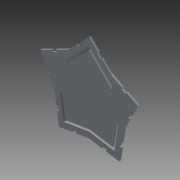
# Autodesk Inventor part: Star Base
Saved by Autodesk Inventor 2015 (Build 190159000, 159)
## iProperties
Created: 2018-03-07
Part Number: Star Base
Material: Generic
Document SubType Name: Modeling
Designer: Administrator
Density: 1 g/cm^3
Appearance: Default
Author: Administrator
Autodesk Inventor part; units mm, degrees
ref_plane "YZ Plane" through (0, 0, 0) normal (1, 0, 0) x (0, 1, 0)
ref_plane "XZ Plane" through (0, 0, 0) normal (0, 1, 0) x (-1, 0, 0)
ref_plane "XY Plane" through (0, 0, 0) normal (0, 0, 1) x (1, 0, 0)
sketch "Sketch1" plane through (0, 0, 0) normal (0, 0, 1) x (1, 0, 0)
  circle A0 centre (0, 0) radius 63.5 construction
  circle A1 centre (0, 0) radius 88.9 construction
  line L0 (0, 88.9) -> (-37.3244, 51.3726)
  line L1 (-37.3244, 51.3726) -> (-84.5489, 27.4716)
  line L2 (-84.5489, 27.4716) -> (-60.3921, -19.6226)
  line L3 (-60.3921, -19.6226) -> (-52.2541, -71.9216)
  line L4 (-52.2541, -71.9216) -> (0, -63.5)
  line L5 (52.2541, -71.9216) -> (0, -63.5)
  line L6 (60.3921, -19.6226) -> (52.2541, -71.9216)
  line L7 (60.3921, -19.6226) -> (84.5489, 27.4716)
  line L8 (84.5489, 27.4716) -> (37.3244, 51.3726)
  line L9 (37.3244, 51.3726) -> (0, 88.9)
  dimension "d0" = 127
  dimension "d1" = 177.8
  dimension "d4" = 360
  dimension "d8" = 360
  constraints: 20 end point, 2 coincident, 2 vertical alignment, 16 other
extrude "Extrusion1" add sketch "Sketch1" along normal blind 3.175
sketch "Sketch2" plane through (0, 0, 3.175) normal (0, 0, 1) x (1, 0, 0)
  line L0 (37.3244, 51.3726) -> (0, 88.9) projected
  line L1 (84.5489, 27.4716) -> (37.3244, 51.3726) projected
  line L2 (60.3921, -19.6226) -> (84.5489, 27.4716) projected
  line L3 (52.2541, -71.9216) -> (60.3921, -19.6226) projected
  line L4 (0, -63.5) -> (52.2541, -71.9216) projected
  line L5 (-21.3489, 67.4349) -> (-19.0978, 65.1959)
  line L6 (-19.0978, 65.1959) -> (-13.7243, 70.5987)
  line L7 (-13.7243, 70.5987) -> (-15.9754, 72.8377)
  line L8 (-21.3489, 67.4349) -> (-15.9754, 72.8377)
  line L9 (0, 70.1363) -> (0, 60.325) construction
  line L10 (21.3489, 67.4349) -> (19.0978, 65.1959)
  line L11 (19.0978, 65.1959) -> (13.7243, 70.5987)
  line L12 (13.7243, 70.5987) -> (15.9754, 72.8377)
  line L13 (21.3489, 67.4349) -> (15.9754, 72.8377)
  line L14 (-64.3361, 37.7016) -> (-62.9023, 34.8688)
  line L15 (-62.9023, 34.8688) -> (-56.1035, 38.3097)
  line L16 (-56.1035, 38.3097) -> (-57.5372, 41.1426)
  line L17 (0, 0) -> (-84.5489, 27.4716) construction
  line L18 (-64.3361, 37.7016) -> (-57.5372, 41.1426)
  line L19 (-74.2094, 7.3145) -> (-71.3844, 8.7636)
  line L20 (-71.3844, 8.7636) -> (-67.9066, 1.9836)
  line L21 (-67.9066, 1.9836) -> (-70.7316, 0.5345)
  line L22 (-74.2094, 7.3145) -> (-70.7316, 0.5345)
  line L23 (-56.9089, -42.0074) -> (-55.7373, -49.5368)
  line L24 (-55.7373, -49.5368) -> (-52.6, -49.0486)
  line L25 (-52.6, -49.0486) -> (-53.7717, -41.5192)
  line L26 (-53.7717, -41.5192) -> (-56.9089, -42.0074)
  line L27 (-52.2541, -71.9216) -> (0, 0) construction
  line L28 (-22.3656, -67.1046) -> (-29.8885, -68.317)
  line L29 (-29.8885, -68.317) -> (-30.3937, -65.1825)
  line L30 (-30.3937, -65.1825) -> (-22.8708, -63.97)
  line L31 (-22.8708, -63.97) -> (-22.3656, -67.1046)
  line L32 (64.3361, 37.7016) -> (62.9023, 34.8688)
  line L33 (62.9023, 34.8688) -> (56.1035, 38.3097)
  line L34 (56.1035, 38.3097) -> (57.5372, 41.1426)
  line L35 (64.3361, 37.7016) -> (57.5372, 41.1426)
  line L36 (71.3844, 8.7636) -> (67.9066, 1.9836)
  line L37 (67.9066, 1.9836) -> (70.7316, 0.5345)
  line L38 (74.2094, 7.3145) -> (70.7316, 0.5345)
  line L39 (74.2094, 7.3145) -> (71.3844, 8.7636)
  line L40 (56.9089, -42.0074) -> (55.7373, -49.5368)
  line L41 (55.7373, -49.5368) -> (52.6, -49.0486)
  line L42 (52.6, -49.0486) -> (53.7717, -41.5192)
  line L43 (53.7717, -41.5192) -> (56.9089, -42.0074)
  line L44 (29.8885, -68.317) -> (30.3937, -65.1825)
  line L45 (22.3656, -67.1046) -> (29.8885, -68.317)
  line L46 (30.3937, -65.1825) -> (22.8708, -63.97)
  line L47 (22.8708, -63.97) -> (22.3656, -67.1046)
  line L48 (-37.3244, 51.3726) -> (-84.5489, 27.4716) projected
  line L49 (0, 88.9) -> (-37.3244, 51.3726) projected
  line L50 (-84.5489, 27.4716) -> (-60.3921, -19.6226) projected
  line L51 (-60.3921, -19.6226) -> (-52.2541, -71.9216) projected
  line L52 (-52.2541, -71.9216) -> (0, -63.5) projected
  point P0 (-18.6622, 70.1363)
  point P1 (18.6622, 70.1363)
  point P2 (60.9366, 39.4221)
  point P3 (72.4705, 3.9245)
  point P4 (56.3231, -45.7721)
  point P5 (-56.3231, -45.7721)
  point P6 (-72.4705, 3.9245)
  point P7 (-60.9366, 39.4221)
  point P8 (-26.1271, -67.7108)
  point P9 (26.1271, -67.7108)
  dimension "d12" = 3.81
  dimension "d13" = 3.81
  dimension "d14" = 3.175
  dimension "d15" = 3.81
  dimension "d16" = 7.62
  dimension "d18" = 3.81
  constraints: 86 end point, 28 symmetric about line, 10 collinear, 5 midpoint, 5 perpendicular, 3 equal length, 1 vertical
  measures "d12" distance from line of L5 point (-18.662, 70.136)
  measures "d13" distance from line of point (-18.662, 70.136) L7
  measures "d14" distance of L6.end L7.end
  measures "d15" distance from line of point (-60.937, 39.422) L14
  measures "d16" distance of L14.end L15.end
  measures "d18" distance from line of L26 point (-56.323, -45.772)
extrude "Extrusion2" cut sketch "Sketch2" against normal blind 25.4 contours L10 L11 L12 L0 | L1 L32 L33 L34 | L7 L6 L5 L8 | L2 L37 L36 L39 | L16 L15 L14 L18 | L3 L41 L42 L43 | L19 L20 L21 L22 | L4 L47 L46 L44 | L26 L25 L24 L23 | L28 L29 L30 L31
sketch "Sketch3" plane through (0, 0, 0) normal (1, 0, 0) x (0, 1, 0)
  line L0 (0, 3.175) -> (0, 185.8962) construction
  line L1 (88.9, 0) -> (88.9, 3.175) projected
  point P0 (0, 0)
  point P1 (0.5345, 3.175)
  dimension "d22" = 88.9
  dimension "d23" = 182.7212
  constraints: 2 end point, 1 vertical
  measures "d22" distance between parallel lines of L1 L0
  measures "d23" distance of L0.start L0.end
sketch "Sketch4" plane through (0, 0, 3.175) normal (0, 0, 1) x (1, 0, 0)
  line L0 (-39.8185, 34.4573) -> (0, 74.4925)
  line L1 (0, 74.4925) -> (39.8185, 34.4573)
  line L2 (39.8185, 34.4573) -> (39.8039, 29.0692)
  line L3 (39.8039, 29.0692) -> (0, 69.0896)
  line L4 (0, 69.0896) -> (-39.8039, 29.0692)
  line L5 (-39.8039, 29.0692) -> (-39.8185, 34.4573)
  line L6 (-21.3489, 67.4349) -> (-37.3244, 51.3726) projected
  line L7 (37.3244, 51.3726) -> (21.3489, 67.4349) projected
  line L8 (-50.5051, -17.0826) -> (-43.7856, -60.2657)
  line L9 (-43.7856, -60.2657) -> (0, -53.2089)
  line L10 (0, -53.2089) -> (43.7856, -60.2657)
  line L11 (43.7856, -60.2657) -> (50.5051, -17.0826)
  line L12 (50.5051, -17.0826) -> (46.1546, -20.2615)
  line L13 (46.1546, -20.2615) -> (40.6099, -55.8947)
  line L14 (40.6099, -55.8947) -> (0, -49.3497)
  line L15 (0, -49.3497) -> (-40.6099, -55.8947)
  line L16 (-40.6099, -55.8947) -> (-46.1546, -20.2615)
  line L17 (-46.1546, -20.2615) -> (-50.5051, -17.0826)
  line L18 (-55.7373, -49.5368) -> (-52.2541, -71.9216) projected
  line L19 (52.2541, -71.9216) -> (55.7373, -49.5368) projected
  line L20 (29.8885, -68.317) -> (52.2541, -71.9216) projected
  line L21 (0, -63.5) -> (22.3656, -67.1046) projected
  line L22 (-22.3656, -67.1046) -> (0, -63.5) projected
  line L23 (-52.2541, -71.9216) -> (-29.8885, -68.317) projected
  line L24 (-37.3244, 51.3726) -> (-57.5372, 41.1426) projected
  point P0 (0, 0)
  point P1 (-60.3921, -19.6226)
  point P2 (60.3921, -19.6226)
  dimension "d24" = 3.81
  dimension "d26" = 10.16
  dimension "d27" = 10.16
  dimension "d29" = 3.81
  dimension "d30" = 2.54
  dimension "d32" = 2.54
  dimension "d33" = 3.81
  dimension "d34" = 3.81
  dimension "d35" = 3.81
  dimension "d36" = 3.81
  dimension "d37" = 10.16
  dimension "d38" = 10.16
  dimension "d39" = 10.16
  dimension "d40" = 10.16
  dimension "d44" = 45
  dimension "d45" = 45
  dimension "d46" = 45
  dimension "d47" = 45
  dimension "d48" = 2.54
  dimension "d50" = 2.54
  constraints: 32 end point, 11 parallel
  measures "d24" distance between parallel lines of L0 L4
  measures "d26" distance between parallel lines of L0 L6
  measures "d27" distance between parallel lines of L7 L1
  measures "d29" distance between parallel lines of L1 L3
  measures "d30" distance from line of L5 L6.end
  measures "d32" distance from line of L2 L7.start
  measures "d33" distance between parallel lines of L16 L8
  measures "d34" distance between parallel lines of L15 L9
  measures "d35" distance between parallel lines of L10 L14
  measures "d36" distance between parallel lines of L11 L13
  measures "d37" distance between parallel lines of L19 L11
  measures "d38" distance between parallel lines of L21 L10
  measures "d39" distance between parallel lines of L23 L9
  measures "d40" distance between parallel lines of L18 L8
  measures "d44" angle of L3 L2
  measures "d45" angle of L4 L5
  measures "d46" angle of L8 L17
  measures "d47" angle of L11 L12
  measures "d48" vertical distance of L8.start point (-60.392, -19.623)
  measures "d50" vertical distance of point (60.392, -19.623) L11.end
extrude "Extrusion3" cut sketch "Sketch4" against normal blind 25.4
body "Solid1"
